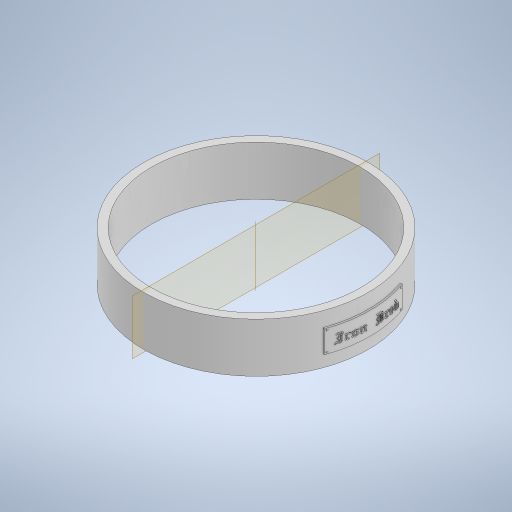
# Autodesk Inventor part: IronDred
Saved by Autodesk Inventor 2023 (Build 270158000, 158)
## iProperties
Created: 2023-04-08
Part Number: IronDred
Material: Generic
Document SubType Name: Modeling
Designer: dntpa
Density: 1 g/cm^3
Appearance: Default
Author: dntpa
## iProperties of the stored document CanisInvictoria_3DPrint.ipt
Created: 2023-04-08
Part Number: CanisInvictoria_3DPrint
Material: Generic
Document SubType Name: Modeling
Designer: dntpa
Density: 1 g/cm^3
Appearance: Default
Author: dntpa
Autodesk Inventor part; units mm, degrees
ref_plane "XZ Plane" through (0, 0, 0) normal (0, 1, 0) x (-1, 0, 0)
ref_plane "XY Plane" through (0, 0, 0) normal (0, 0, 1) x (1, 0, 0)
sketch "Sketch1" plane through (0, 0, 0) normal (0, 1, 0) x (-1, 0, 0)
  circle A0 centre (0, 0) radius 50
  circle A1 centre (0, 0) radius 46.5
  dimension "d0" = 100
  dimension "d1" = 93
  constraints: 2 centre point, 2 coincident
  measures "d0" diameter of A0
  measures "d1" diameter of A1
extrude "Extrusion1" add sketch "Sketch1" along normal blind 22
ref_plane "Work Plane1" through (60, 0, 0) normal (1, 0, 0) x (0, 1, 0)
sketch "Text" plane through (60, 0, 0) normal (1, 0, 0) x (0, 1, 0)
  line L0 (15.4535, 17.5) -> (15.4535, -17.5) construction
  line L1 (15.4535, -17.5) -> (5.4535, -17.5) construction
  line L2 (5.4535, -17.5) -> (5.4535, 17.5) construction
  line L3 (5.4535, 17.5) -> (15.4535, 17.5) construction
  line L4 (22, -50) -> (22, 50) projected
  line L5 (5.4535, 17.5) -> (15.4535, 17.5)
  line L6 (15.4535, 17.5) -> (15.4535, -17.5)
  line L7 (15.4535, -17.5) -> (5.4535, -17.5)
  line L8 (5.4535, -17.5) -> (5.4535, 17.5)
  line L9 (15.4535, 17.5) -> (15.4535, 0)
  line L10 (15.4535, 0) -> (15.4535, -17.5)
  circle A0 centre (14.7035, 16.75) radius 0.375
  line L11 (22, 0) -> (0, 0)
  line L12 (10.4535, 17.5) -> (10.4535, -17.5)
  circle A1 centre (14.7035, -16.75) radius 0.375
  circle A2 centre (6.2035, 16.75) radius 0.375
  circle A3 centre (6.2035, -16.75) radius 0.375
  line L13 (12.1974, 11.0153) -> (11.6167, 11.3039)
  line L14 (11.6167, 11.3039) -> (9.4453, 11.3039)
  line L15 (9.4453, 11.3039) -> (9.0666, 11.4878)
  spline S0 degree 2 poles (9.0666, 11.4878) (8.9945, 11.56) (8.8141, 11.7439) (8.7059, 11.8521) knots 0 0 0 1 2 2 2
  line L16 (8.7059, 11.8521) -> (8.6915, 11.8593)
  line L17 (8.6915, 11.8593) -> (8.6915, 11.8774)
  line L18 (8.6915, 11.8774) -> (8.5112, 12.2381)
  line L19 (8.5112, 12.2381) -> (8.5112, 12.8007)
  line L20 (8.5112, 12.8007) -> (8.6915, 13.165)
  line L21 (8.6915, 13.165) -> (8.6915, 13.6844)
  line L22 (8.6915, 13.6844) -> (8.4066, 14.2687)
  line L23 (8.4066, 14.2687) -> (8.7636, 13.9044)
  spline S1 degree 2 poles (8.7636, 13.9044) (8.7961, 13.8792) (8.8863, 13.7854) (8.9476, 13.7205) knots 0 0 0 1 2 2 2
  line L24 (8.9476, 13.7205) -> (9.1351, 13.3454)
  line L25 (9.1351, 13.3454) -> (9.1351, 12.963)
  line L26 (9.1351, 12.963) -> (8.7709, 12.2381)
  line L27 (8.7709, 12.2381) -> (8.7709, 11.9098)
  line L28 (8.7709, 11.9098) -> (9.1063, 11.7475)
  line L29 (9.1063, 11.7475) -> (11.0901, 11.7475)
  spline S2 degree 2 poles (11.0901, 11.7475) (11.2199, 11.7042) (11.494, 11.6105) (11.6455, 11.56) knots 0 0 0 1 2 2 2
  line L30 (11.6455, 11.56) -> (12.1974, 11.0153)
  spline S3 degree 2 poles (9.99, 12.2056) (9.9106, 12.2417) (9.7231, 12.3354) (9.6113, 12.3931) knots 0 0 0 1 2 2 2
  spline S4 degree 2 poles (9.6113, 12.3931) (9.5608, 12.4436) (9.4381, 12.5699) (9.3588, 12.6492) knots 0 0 0 1 2 2 2
  line L31 (9.3588, 12.6492) -> (10.3218, 12.6492)
  line L32 (10.3218, 12.6492) -> (10.3218, 12.9558)
  line L33 (10.3218, 12.9558) -> (10.0838, 13.1939)
  line L34 (10.0838, 13.1939) -> (10.5562, 13.1939)
  line L35 (10.5562, 13.1939) -> (10.7654, 12.9847)
  line L36 (10.7654, 12.9847) -> (10.7654, 12.6492)
  line L37 (10.7654, 12.6492) -> (10.9133, 12.6492)
  spline S5 degree 2 poles (10.9133, 12.6492) (10.9963, 12.6132) (11.1802, 12.5194) (11.292, 12.4617) knots 0 0 0 1 2 2 2
  spline S6 degree 2 poles (11.292, 12.4617) (11.3425, 12.4112) (11.4652, 12.2849) (11.5445, 12.2056) knots 0 0 0 1 2 2 2
  line L38 (11.5445, 12.2056) -> (9.99, 12.2056)
  line L39 (12.5003, 11.4914) -> (11.9485, 12.0505)
  line L40 (11.9485, 12.0505) -> (11.9485, 12.6168)
  line L41 (11.9485, 12.6168) -> (12.1252, 13.147)
  line L42 (12.1252, 13.147) -> (11.8403, 13.7241)
  line L43 (11.8403, 13.7241) -> (12.3921, 13.1686)
  line L44 (12.3921, 13.1686) -> (12.3921, 12.606)
  spline S7 degree 2 poles (12.3921, 12.606) (12.3705, 12.5338) (12.2803, 12.2705) (12.2154, 12.0721) knots 0 0 0 1 2 2 2
  line L45 (12.2154, 12.0721) -> (12.5003, 11.4914)
  line L46 (10.7654, 7.8774) -> (10.4985, 8.4076)
  line L47 (10.4985, 8.4076) -> (10.4985, 8.7935)
  line L48 (10.4985, 8.7935) -> (10.852, 9.1506)
  line L49 (10.852, 9.1506) -> (10.6969, 9.4608)
  line L50 (10.6969, 9.4608) -> (9.1207, 9.4608)
  line L51 (9.1207, 9.4608) -> (8.9548, 9.1289)
  line L52 (8.9548, 9.1289) -> (8.9548, 8.7827)
  line L53 (8.9548, 8.7827) -> (8.7853, 9.1253)
  spline S8 degree 2 poles (8.7853, 9.1253) (8.7636, 9.1614) (8.7204, 9.248) (8.6951, 9.2949) knots 0 0 0 1 2 2 2
  spline S9 degree 2 poles (8.6951, 9.2949) (8.6843, 9.3093) (8.4967, 9.5005) knots 0 0 0 1 1 1
  spline S10 degree 2 poles (8.4967, 9.5005) (8.6771, 9.6844) (8.7131, 9.7421) knots 0 0 0 1 1 1
  spline S11 degree 2 poles (8.7131, 9.7421) (8.7168, 9.7457) (8.7925, 9.9008) (8.8718, 10.0523) knots 0 0 0 1 2 2 2
  line L54 (8.8718, 10.0523) -> (8.8718, 10.4022)
  line L55 (8.8718, 10.4022) -> (9.1207, 9.9044)
  line L56 (9.1207, 9.9044) -> (10.5274, 9.9044)
  line L57 (10.5274, 9.9044) -> (10.6825, 10.0595)
  line L58 (10.6825, 10.0595) -> (10.6825, 10.3228)
  line L59 (10.6825, 10.3228) -> (11.1406, 9.8647)
  line L60 (11.1406, 9.8647) -> (10.7727, 9.4896)
  line L61 (10.7727, 9.4896) -> (11.137, 8.7683)
  spline S12 degree 2 poles (11.137, 8.7683) (11.0865, 8.7214) (10.9927, 8.624) (10.9422, 8.5735) knots 0 0 0 1 2 2 2
  spline S13 degree 2 poles (10.9422, 8.5735) (10.935, 8.5627) (10.7654, 8.2236) knots 0 0 0 1 1 1
  line L62 (10.7654, 8.2236) -> (10.7654, 7.8774)
  line L63 (10.7654, 4.9522) -> (10.5202, 5.4463)
  line L64 (10.5202, 5.4463) -> (8.8718, 5.4463)
  line L65 (8.8718, 5.4463) -> (8.8718, 5.8467)
  spline S14 degree 2 poles (8.8718, 5.8467) (8.8682, 5.8611) (8.843, 5.9477) (8.8177, 6.0234) knots 0 0 0 1 2 2 2
  line L66 (8.8177, 6.0234) -> (8.6987, 6.3769)
  spline S15 degree 2 poles (8.6987, 6.3769) (8.6627, 6.4418) (8.5689, 6.6366) (8.5039, 6.7665) knots 0 0 0 1 2 2 2
  line L67 (8.5039, 6.7665) -> (8.6987, 6.9612)
  spline S16 degree 2 poles (8.6987, 6.9612) (8.76, 7.0947) (8.8718, 7.3111) knots 0 0 0 1 1 1
  line L68 (8.8718, 7.3111) -> (8.8718, 7.8377)
  line L69 (8.8718, 7.8377) -> (9.1207, 7.3399)
  line L70 (9.1207, 7.3399) -> (10.7654, 7.3399)
  line L71 (10.7654, 7.3399) -> (10.7654, 6.9396)
  spline S17 degree 2 poles (10.7654, 6.9396) (10.7727, 6.9288) (10.7979, 6.8386) (10.8232, 6.7665) knots 0 0 0 1 2 2 2
  line L72 (10.8232, 6.7665) -> (10.9422, 6.4094)
  spline S18 degree 2 poles (10.9422, 6.4094) (10.9746, 6.3408) (11.072, 6.1497) (11.137, 6.0234) knots 0 0 0 1 2 2 2
  spline S19 degree 2 poles (11.137, 6.0234) (11.0901, 5.9729) (10.9927, 5.8756) (10.9422, 5.8251) knots 0 0 0 1 2 2 2
  spline S20 degree 2 poles (10.9422, 5.8251) (10.935, 5.8142) (10.8484, 5.6447) (10.7654, 5.4788) knots 0 0 0 1 2 2 2
  line L73 (10.7654, 5.4788) -> (10.7654, 4.9522)
  line L74 (8.944, 5.89) -> (10.5166, 5.89)
  spline S21 degree 2 poles (10.5166, 5.89) (10.5454, 5.9585) (10.632, 6.1317) (10.6861, 6.2399) knots 0 0 0 1 2 2 2
  spline S22 degree 2 poles (10.6861, 6.2399) (10.7258, 6.2759) (10.8087, 6.3589) (10.8592, 6.4022) knots 0 0 0 1 2 2 2
  line L75 (10.8592, 6.4022) -> (10.6933, 6.8963)
  line L76 (10.6933, 6.8963) -> (9.1207, 6.8963)
  spline S23 degree 2 poles (9.1207, 6.8963) (9.0919, 6.8314) (9.0053, 6.6546) (8.9512, 6.55) knots 0 0 0 1 2 2 2
  line L77 (8.9512, 6.55) -> (8.7781, 6.3841)
  line L78 (8.7781, 6.3841) -> (8.944, 5.89)
  line L79 (10.7654, 1.6628) -> (10.5166, 2.1569)
  line L80 (10.5166, 2.1569) -> (9.1099, 2.1569)
  line L81 (9.1099, 2.1569) -> (8.9548, 2.0018)
  line L82 (8.9548, 2.0018) -> (8.9548, 1.7385)
  line L83 (8.9548, 1.7385) -> (8.4967, 2.2002)
  line L84 (8.4967, 2.2002) -> (8.8971, 2.6005)
  line L85 (8.8971, 2.6005) -> (10.5166, 2.6005)
  line L86 (10.5166, 2.6005) -> (10.6789, 2.936)
  line L87 (10.6789, 2.936) -> (10.6789, 3.0983)
  line L88 (10.6789, 3.0983) -> (10.5094, 3.6069)
  line L89 (10.5094, 3.6069) -> (9.1207, 3.6069)
  line L90 (9.1207, 3.6069) -> (8.9223, 3.2137)
  line L91 (8.9223, 3.2137) -> (8.4967, 3.6465)
  spline S24 degree 2 poles (8.4967, 3.6465) (8.6771, 3.8305) (8.7131, 3.8882) knots 0 0 0 1 1 1
  spline S25 degree 2 poles (8.7131, 3.8882) (8.7168, 3.8918) (8.7925, 4.0469) (8.8718, 4.1984) knots 0 0 0 1 2 2 2
  line L92 (8.8718, 4.1984) -> (8.8718, 4.5482)
  line L93 (8.8718, 4.5482) -> (9.1207, 4.0505)
  line L94 (9.1207, 4.0505) -> (10.5274, 4.0505)
  line L95 (10.5274, 4.0505) -> (10.6825, 4.2056)
  line L96 (10.6825, 4.2056) -> (10.6825, 4.4689)
  line L97 (10.6825, 4.4689) -> (11.1406, 4.0108)
  line L98 (11.1406, 4.0108) -> (10.7402, 3.6069)
  line L99 (10.7402, 3.6069) -> (10.5959, 3.6069)
  spline S26 degree 2 poles (10.5959, 3.6069) (10.6176, 3.5203) (10.7005, 3.2786) (10.7582, 3.1199) knots 0 0 0 1 2 2 2
  line L100 (10.7582, 3.1199) -> (10.8773, 2.8855)
  spline S27 degree 2 poles (10.8773, 2.8855) (10.8917, 2.853) (10.9422, 2.7665) knots 0 0 0 1 1 1
  spline S28 degree 2 poles (10.9422, 2.7665) (10.953, 2.752) (11.1406, 2.5609) knots 0 0 0 1 1 1
  spline S29 degree 2 poles (11.1406, 2.5609) (10.9602, 2.3805) (10.9205, 2.3156) knots 0 0 0 1 1 1
  spline S30 degree 2 poles (10.9205, 2.3156) (10.9025, 2.2976) (10.7654, 2.009) knots 0 0 0 1 1 1
  line L101 (10.7654, 2.009) -> (10.7654, 1.6628)
  line L102 (9.0522, -5.8647) -> (9.0522, -5.4716)
  line L103 (9.0522, -5.4716) -> (8.8755, -5.1253)
  line L104 (8.8755, -5.1253) -> (8.5039, -4.7502)
  line L105 (8.5039, -4.7502) -> (8.6915, -4.3643)
  line L106 (8.6915, -4.3643) -> (8.6915, -3.477)
  spline S31 degree 2 poles (8.6915, -3.477) (8.6735, -3.4121) (8.5581, -2.9396) (8.4571, -2.5248) knots 0 0 0 1 2 2 2
  line L107 (8.4571, -2.5248) -> (8.6194, -2.7737)
  line L108 (8.6194, -2.7737) -> (8.9476, -3.2714)
  line L109 (8.9476, -3.2714) -> (9.1351, -3.8269)
  line L110 (9.1351, -3.8269) -> (9.1351, -4.3354)
  line L111 (9.1351, -4.3354) -> (11.9485, -4.3354)
  line L112 (11.9485, -4.3354) -> (11.9485, -3.2822)
  spline S32 degree 2 poles (11.9485, -3.2822) (11.9846, -3.1993) (12.0783, -3.0117) (12.136, -2.9035) knots 0 0 0 1 2 2 2
  spline S33 degree 2 poles (12.136, -2.9035) (12.1865, -2.853) (12.3128, -2.7268) (12.3921, -2.651) knots 0 0 0 1 2 2 2
  line L113 (12.3921, -2.651) -> (12.3921, -5.2913)
  line L114 (12.3921, -5.2913) -> (12.201, -5.6736)
  line L115 (12.201, -5.6736) -> (11.8186, -5.8647)
  line L116 (11.8186, -5.8647) -> (9.0522, -5.8647)
  line L117 (9.1207, -5.4211) -> (9.9719, -5.4211)
  line L118 (9.9719, -5.4211) -> (10.1379, -5.0929)
  line L119 (10.1379, -5.0929) -> (10.1379, -4.7502)
  line L120 (10.1379, -4.7502) -> (9.9719, -4.422)
  line L121 (9.9719, -4.422) -> (9.1351, -4.422)
  line L122 (9.1351, -4.422) -> (9.1351, -4.5663)
  spline S34 degree 2 poles (9.1351, -4.5663) (9.1315, -4.5699) (9.0486, -4.8368) (8.9584, -5.0965) knots 0 0 0 1 2 2 2
  line L123 (8.9584, -5.0965) -> (9.1207, -5.4211)
  spline S35 degree 2 poles (9.99, -3.8774) (9.9106, -3.8413) (9.7231, -3.7511) (9.6113, -3.6934) knots 0 0 0 1 2 2 2
  spline S36 degree 2 poles (9.6113, -3.6934) (9.5608, -3.6429) (9.4381, -3.5131) (9.3588, -3.4337) knots 0 0 0 1 2 2 2
  line L124 (9.3588, -3.4337) -> (10.3218, -3.4337)
  line L125 (10.3218, -3.4337) -> (10.3218, -3.1307)
  line L126 (10.3218, -3.1307) -> (10.0838, -2.8891)
  line L127 (10.0838, -2.8891) -> (10.5562, -2.8891)
  line L128 (10.5562, -2.8891) -> (10.7654, -3.0947)
  line L129 (10.7654, -3.0947) -> (10.7654, -3.4337)
  line L130 (10.7654, -3.4337) -> (10.9133, -3.4337)
  spline S37 degree 2 poles (10.9133, -3.4337) (10.9963, -3.4698) (11.1802, -3.56) (11.292, -3.6177) knots 0 0 0 1 2 2 2
  spline S38 degree 2 poles (11.292, -3.6177) (11.3425, -3.6682) (11.4652, -3.798) (11.5445, -3.8774) knots 0 0 0 1 2 2 2
  line L131 (11.5445, -3.8774) -> (9.99, -3.8774)
  line L132 (11.1117, -5.4211) -> (11.7934, -5.4211)
  line L133 (11.7934, -5.4211) -> (11.9485, -5.266)
  line L134 (11.9485, -5.266) -> (11.9485, -4.422)
  line L135 (11.9485, -4.422) -> (11.1117, -4.422)
  line L136 (11.1117, -4.422) -> (10.9458, -4.7538)
  line L137 (10.9458, -4.7538) -> (10.9458, -5.0929)
  line L138 (10.9458, -5.0929) -> (11.1117, -5.4211)
  line L139 (10.0657, -5.4211) -> (11.0179, -5.4211)
  line L140 (11.0179, -5.4211) -> (10.8628, -5.1109)
  line L141 (10.8628, -5.1109) -> (10.8628, -4.7286)
  line L142 (10.8628, -4.7286) -> (11.0179, -4.422)
  line L143 (11.0179, -4.422) -> (10.0657, -4.422)
  line L144 (10.0657, -4.422) -> (10.2208, -4.7286)
  line L145 (10.2208, -4.7286) -> (10.2208, -5.1109)
  line L146 (10.2208, -5.1109) -> (10.0657, -5.4211)
  line L147 (10.7654, -9.2876) -> (10.4985, -8.7574)
  line L148 (10.4985, -8.7574) -> (10.4985, -8.3715)
  line L149 (10.4985, -8.3715) -> (10.852, -8.0144)
  line L150 (10.852, -8.0144) -> (10.6969, -7.7042)
  line L151 (10.6969, -7.7042) -> (9.1207, -7.7042)
  line L152 (9.1207, -7.7042) -> (8.9548, -8.0361)
  line L153 (8.9548, -8.0361) -> (8.9548, -8.3823)
  line L154 (8.9548, -8.3823) -> (8.7853, -8.0397)
  spline S39 degree 2 poles (8.7853, -8.0397) (8.7636, -8.0036) (8.7204, -7.917) (8.6951, -7.8702) knots 0 0 0 1 2 2 2
  spline S40 degree 2 poles (8.6951, -7.8702) (8.6843, -7.8557) (8.4967, -7.6646) knots 0 0 0 1 1 1
  spline S41 degree 2 poles (8.4967, -7.6646) (8.6771, -7.4806) (8.7131, -7.4229) knots 0 0 0 1 1 1
  spline S42 degree 2 poles (8.7131, -7.4229) (8.7168, -7.4193) (8.7925, -7.2642) (8.8718, -7.1127) knots 0 0 0 1 2 2 2
  line L155 (8.8718, -7.1127) -> (8.8718, -6.7628)
  line L156 (8.8718, -6.7628) -> (9.1207, -7.2606)
  line L157 (9.1207, -7.2606) -> (10.5274, -7.2606)
  line L158 (10.5274, -7.2606) -> (10.6825, -7.1055)
  line L159 (10.6825, -7.1055) -> (10.6825, -6.8422)
  line L160 (10.6825, -6.8422) -> (11.1406, -7.3003)
  line L161 (11.1406, -7.3003) -> (10.7727, -7.6754)
  line L162 (10.7727, -7.6754) -> (11.137, -8.3968)
  spline S43 degree 2 poles (11.137, -8.3968) (11.0865, -8.4436) (10.9927, -8.541) (10.9422, -8.5915) knots 0 0 0 1 2 2 2
  spline S44 degree 2 poles (10.9422, -8.5915) (10.935, -8.6023) (10.7654, -8.9414) knots 0 0 0 1 1 1
  line L163 (10.7654, -8.9414) -> (10.7654, -9.2876)
  line L164 (10.3507, -11.5564) -> (9.6113, -10.2687)
  line L165 (9.6113, -10.2687) -> (9.1207, -10.2687)
  line L166 (9.1207, -10.2687) -> (8.9548, -10.6005)
  line L167 (8.9548, -10.6005) -> (8.9548, -10.9468)
  line L168 (8.9548, -10.9468) -> (8.7853, -10.6041)
  spline S45 degree 2 poles (8.7853, -10.6041) (8.7636, -10.5681) (8.7204, -10.4815) (8.6951, -10.4346) knots 0 0 0 1 2 2 2
  spline S46 degree 2 poles (8.6951, -10.4346) (8.6843, -10.4202) (8.4967, -10.229) knots 0 0 0 1 1 1
  spline S47 degree 2 poles (8.4967, -10.229) (8.6771, -10.0451) (8.7131, -9.9874) knots 0 0 0 1 1 1
  spline S48 degree 2 poles (8.7131, -9.9874) (8.7168, -9.9838) (8.7925, -9.8287) (8.8718, -9.6772) knots 0 0 0 1 2 2 2
  line L169 (8.8718, -9.6772) -> (8.8718, -9.3273)
  line L170 (8.8718, -9.3273) -> (9.1207, -9.8251)
  line L171 (9.1207, -9.8251) -> (10.7546, -9.8251)
  line L172 (10.7546, -9.8251) -> (10.9458, -10.5753)
  spline S49 degree 2 poles (10.9458, -10.5753) (10.953, -10.5969) (11.137, -10.9612) knots 0 0 0 1 1 1
  line L173 (11.137, -10.9612) -> (10.3507, -11.5564)
  line L174 (10.1739, -11.0875) -> (10.852, -10.5789)
  line L175 (10.852, -10.5789) -> (10.6969, -10.2687)
  line L176 (10.6969, -10.2687) -> (9.7086, -10.2687)
  line L177 (9.7086, -10.2687) -> (10.1739, -11.0875)
  line L178 (8.8718, -14.2831) -> (8.8718, -13.8828)
  spline S50 degree 2 poles (8.8718, -13.8828) (8.8682, -13.8683) (8.843, -13.7818) (8.8177, -13.706) knots 0 0 0 1 2 2 2
  line L179 (8.8177, -13.706) -> (8.6987, -13.3526)
  spline S51 degree 2 poles (8.6987, -13.3526) (8.6627, -13.2876) (8.5689, -13.0929) (8.5039, -12.963) knots 0 0 0 1 2 2 2
  line L180 (8.5039, -12.963) -> (8.6987, -12.7683)
  spline S52 degree 2 poles (8.6987, -12.7683) (8.76, -12.6348) (8.8718, -12.4184) knots 0 0 0 1 1 1
  line L181 (8.8718, -12.4184) -> (8.8718, -11.8918)
  line L182 (8.8718, -11.8918) -> (9.1207, -12.3895)
  line L183 (9.1207, -12.3895) -> (10.7546, -12.3895)
  line L184 (10.7546, -12.3895) -> (10.8159, -12.5807)
  line L185 (10.8159, -12.5807) -> (10.9422, -12.9594)
  line L186 (10.9422, -12.9594) -> (11.0973, -13.2624)
  line L187 (11.0973, -13.2624) -> (11.9954, -12.3643)
  line L188 (11.9954, -12.3643) -> (12.4138, -12.9955)
  line L189 (12.4138, -12.9955) -> (11.8295, -13.1939)
  line L190 (11.8295, -13.1939) -> (10.7402, -14.2831)
  line L191 (10.7402, -14.2831) -> (8.8718, -14.2831)
  line L192 (8.944, -13.8395) -> (10.5274, -13.8395)
  line L193 (10.5274, -13.8395) -> (11.0324, -13.3309)
  line L194 (11.0324, -13.3309) -> (10.7005, -12.8332)
  line L195 (10.7005, -12.8332) -> (9.1207, -12.8332)
  spline S53 degree 2 poles (9.1207, -12.8332) (9.0919, -12.8981) (9.0053, -13.0748) (8.9512, -13.1794) knots 0 0 0 1 2 2 2
  line L196 (8.9512, -13.1794) -> (8.7781, -13.3454)
  line L197 (8.7781, -13.3454) -> (8.944, -13.8395)
  dimension "d6" = 11.5465
  dimension "d10" = 0
  dimension "d11" = 10
  dimension "d12" = 35
  dimension "d25" = 0.75
  dimension "d26" = 0.75
  dimension "d27" = 0.75
  constraints: 16 end point, 5 midpoint, 4 centre point, 3 symmetric about line, 2 collinear, 2 horizontal, 2 parallel, 1 perpendicular, 5 other
  measures "d6" distance from line of L4 L12.start
  measures "d10" vertical distance of L11.start point (15.453, 0)
  measures "d11" distance between parallel lines of L0 L2
  measures "d12" distance between parallel lines of L3 L1
  measures "d25" diameter of A0
  measures "d26" distance from line of L0 A0.centre
  measures "d27" distance from line of L3 A0.centre
sketch "NamePlate" plane through (60, 0, 0) normal (1, 0, 0) x (0, 1, 0)
  line L0 (15.4535, 17.5) -> (5.4535, 17.5)
  line L1 (5.4535, 17.5) -> (5.4535, -17.5)
  line L2 (5.4535, -17.5) -> (15.4535, -17.5)
  line L3 (15.4535, -17.5) -> (15.4535, 17.5)
  point P0 (0, 0)
  point P1 (15.4535, 17.5)
  point P2 (5.4535, -17.5)
  dimension "d19" = 0
  dimension "d20" = 0
  constraints: 8 end point, 2 parallel, 1 horizontal, 1 perpendicular
  measures "d19" distance from line of point (15.453, 17.5) L0
  measures "d20" distance from line of point (5.453, -17.5) L2
emboss "Emboss4" sketch "NamePlate" operation add depth 0.75 direction (1, 0, 0) wrap yes faces at (32.9673, 14.6667, 37.592)
emboss "Emboss5" sketch "Text" operation add depth 0.5 direction (1, 0, 0) wrap yes faces at (50.6853, 8.7868, 2.5615) contours L34 L35 L36 L37 S5 S6 L38 L12 | L12 L38 S3 S4 L31 L32 L33 L34 | L80 L81 L82 L83 L84 L85 L12 | L12 L85 L86 L87 L88 L89 L94 L95 L96 L97 L98 L99 S26 L100 S27 S28 S29 S30 L101 L79 L80 | L127 L128 L129 L130 S37 S38 L131 L12 | L12 L131 S35 S36 L124 L125 L126 L127 | L29 S2 L30 L13 L14 L12 | L12 L14 L15 S0 L16 L17 L18 L19 L20 L21 L22 L23 S1 L24 L25 L26 L27 L28 L29 | L191 L178 S50 L179 S51 L180 S52 L181 L182 L183 L12 L195 S53 L196 L197 L192 | L12 L192 L193 L194 L195 L183 L184 L185 L186 L187 L188 L189 L190 L191 | L89 L90 L91 S24 S25 L92 L93 L94 L12 | L111 L112 S32 S33 L113 L114 L115 L116 L12 L139 L140 L141 L142 L143 | L12 L143 L144 L145 L146 L139 L116 L102 L103 L104 L105 L106 S31 L107 L108 L109 L110 L111 | L56 L57 L58 L59 L60 L61 S12 S13 L62 L46 L47 L48 L49 L50 L12 | L12 L50 L51 L52 L53 S8 S9 S10 S11 L54 L55 L56 | L64 L65 S14 L66 S15 L67 S16 L68 L69 L70 L12 L76 S23 L77 L78 L74 | L12 L74 S21 S22 L75 L76 L70 L71 S17 L72 S18 S19 S20 L73 L63 L64 | L173 L164 L165 L166 L167 L168 S45 S46 S47 S48 L169 L170 L171 L12 L176 L177 L174 | L12 L174 L175 L176 L171 L172 S49 L173 | L157 L158 L159 L160 L161 L162 S43 S44 L163 L147 L148 L149 L150 L151 L12 | L12 L151 L152 L153 L154 S39 S40 S41 S42 L155 L156 L157 | L39 L40 L41 L42 L43 L44 S7 L45
emboss "Emboss6" sketch "Text" operation add depth 0.4 direction (1, 0, 0) wrap yes faces at (48.0599, 9.7712, 16.3036) contours A0 | A1 | A2 | A3
fillet "Rivots" radius 0.35 4 edges at (48.3892, 14.3285, 16.5772) (48.3892, 5.8285, 16.5772) (48.3892, 14.3285, -16.5772) (48.3892, 5.8285, -16.5772)
pattern_circular "Circular Pattern1" count 2 over 360 about axis through (0, -10, 0) along (0, 1, 0) of "Emboss4"
pattern_circular "Circular Pattern2" count 2 over 360 about axis through (0, -10, 0) along (0, 1, 0) of "Emboss5"
pattern_circular "Circular Pattern3" count 2 over 360 about axis through (0, -10, 0) along (0, 1, 0) of "Emboss6"
body "Solid1"
